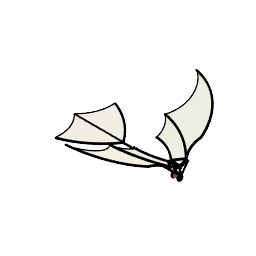
Ornithopter full model (Autodesk Fusion 360 design; units mm, degrees)
Autodesk Fusion 360 part; units mm, degrees
sketch "Sketch1" plane through (0, 0, 0) normal (1, 0, 0) x (0, 1, 0) in component "Component"
  circle A0 centre (0, 0) radius 5
  line L0 (-1, 6.9282) -> (-1, 25)
  arc A1 (1, 25) -> (-1, 25) centre (0, 25) ccw
  line L1 (1, 25) -> (1, 6.9282)
  arc A2 (-1, 6.9282) -> (1, 6.9282) centre (0, 0) ccw
  dimension "d1" = 10
  dimension "d3" = 7
  dimension "d4" = 25
  dimension "d5" = 1
  constraint coincident A0.centre A2.centre
  constraint vertical L0
  constraint tangent L0 A1
  constraint tangent A1 L1
  constraint parallel L0 L1
  constraint concentric A0 A2
  constraint vertical A0.centre A1.centre
  measures "d1" diameter of A0
  measures "d3" radius of A2
  measures "d4" distance of A0.centre A1.centre
  measures "d5" radius of A1
extrude "Extrude1" add sketch "Sketch1" against normal blind 2 makes body 1 in component "Component"
sketch "Sketch2" plane through (0, 0, 0) normal (1, 0, 0) x (0, 1, 0) in component "Component"
  circle A0 centre (0, 0) radius 5
  arc A1 (1, 25) -> (-1, 25) centre (0, 25) ccw
  line L0 (-1, 25) -> (-1, 6.9282)
  arc A2 (-1, 6.9282) -> (1, 6.9282) centre (0, 0) ccw
  line L1 (1, 6.9282) -> (1, 25)
  circle A3 centre (0, 25) radius 1
  dimension "d8" = 2
  constraint concentric A1 A3
  measures "d8" diameter of A3
extrude "Extrude2" add sketch "Sketch2" along normal blind 2 and the other way blind 30 contours A1 A3 bodies 1 in component "Component"
sketch "Sketch3" plane through (-2, 0, 0) normal (-1, 0, 0) x (0, -1, 0) in component "Component"
  arc A0 (-1, 25) -> (1, 25) centre (0, 25) ccw
  line L0 (-1, 25) -> (-1, 6.9282)
  arc A1 (-1, 6.9282) -> (1, 6.9282) centre (0, 0) ccw
  line L1 (1, 6.9282) -> (1, 25)
  circle A2 centre (0, 0) radius 5
  line L2 (1, 7) -> (-1, 7)
  line L3 (-1, 7) -> (-1, 5)
  line L4 (-1, 5) -> (1, 5)
  line L5 (1, 5) -> (1, 7)
  line L6 (1, 7) -> (-1, 5) construction
  line L7 (-1, 7) -> (1, 5) construction
  point P0 (0, 6)
  dimension "d13" = 2
  dimension "d14" = 2
  constraint horizontal L2
  constraint perpendicular L2 L3
  constraint parallel L2 L4
  constraint parallel L3 L5
  constraint coincident L6 P0
  constraint coincident L7 P0
  constraint coincident L1 L2.start
  constraint tangent A2 L4
  measures "d13" distance of L2.start L2.end
  measures "d14" distance of L2.start L4.end
extrude "Extrude4" add sketch "Sketch3" along normal blind 146 contours L0 L1 L2 L3 L4 L5 bodies 1 in component "Component"
ref_plane "WorkPlane1" through (-16, 0, 9) normal (1, 0, 0) x (0, 1, 0) in component "Component"
sketch "Sketch4" plane through (-16, 0, 0) normal (1, 0, 0) x (0, 1, 0) in component "Component"
  circle A0 centre (0, 0) radius 5
  circle A1 centre (0, 0) radius 7
  dimension "d20" = 2
extrude "Extrude5" add sketch "Sketch4" against normal blind 2 bodies 1 in component "Component"
sketch "Sketch5" plane through (-148, 0, 0) normal (-1, 0, 0) x (0, -1, 0) in component "Component"
  line L0 (1, 5) -> (1, 7)
  line L1 (1, 7) -> (-1, 7)
  line L2 (-1, 7) -> (-1, 5)
  line L3 (-1, 5) -> (1, 5)
  line L4 (0.512, 5.5) -> (-0.488, 5.5)
  line L5 (-0.488, 5.5) -> (-0.488, 6.5)
  line L6 (-0.488, 6.5) -> (0.512, 6.5)
  line L7 (0.512, 6.5) -> (0.512, 5.5)
  line L8 (0.512, 5.5) -> (-0.488, 6.5) construction
  line L9 (-0.488, 5.5) -> (0.512, 6.5) construction
  line L10 (1, 7) -> (-1, 7)
  point P0 (0.012, 6)
  dimension "d23" = 1
  dimension "d24" = 1
  dimension "d25" = 0.5
  constraint horizontal L4
  constraint perpendicular L4 L5
  constraint parallel L4 L6
  constraint parallel L5 L7
  constraint coincident L8 P0
  constraint coincident L9 P0
  measures "d23" distance of L4.end L5.end
  measures "d24" distance of L5.end L6.end
  measures "d25" distance of L6 L10
extrude "Extrude6" add sketch "Sketch5" along normal blind 0.7 contours L4 L5 L6 L7 bodies 1 in component "Component"
ref_plane "WorkPlane2" through (-98, 0, -0.0359) normal (-1, 0, 0) x (0, -1, 0) in component "Component"
sketch "Sketch6" plane through (-98, 0, 0) normal (-1, 0, 0) x (0, -1, 0) in component "Component"
  line L0 (-1, 7) -> (1, 7)
  line L1 (1, 7) -> (1, 9)
  line L2 (1, 9) -> (-1, 9)
  line L3 (-1, 9) -> (-1, 7)
  line L4 (-1, 7) -> (1, 9) construction
  line L5 (1, 7) -> (-1, 9) construction
  line L6 (1, 7) -> (-1, 7)
  point P0 (0, 8)
  dimension "d29" = 2
  dimension "d30" = 2
  constraint horizontal L0
  constraint perpendicular L0 L1
  constraint parallel L0 L2
  constraint parallel L1 L3
  constraint coincident L4 P0
  constraint coincident L5 P0
  constraint vertical P0 origin
  constraint collinear L0 L6
  measures "d29" distance of L1.end L2.end
  measures "d30" distance of L0.start L2.end
extrude "Extrude7" add sketch "Sketch6" along normal blind 2 bodies 1 in component "Component"
sketch "Sketch2 (2)" plane through (0, 0, 0) normal (1, 0, 0) x (0, 1, 0) in component "Component'"
  circle A0 centre (0, 0) radius 5
  dimension "d36" = 10
  constraint coincident A0.centre origin
  measures "d36" diameter of A0
extrude "Extrude2'" add sketch "Sketch2 (2)" against normal blind 20 separate body makes body 2 in component "Component'"
sketch "Sketch3 (2)" plane through (0, 0, 0) normal (1, 0, 0) x (0, 1, 0) in component "Component'"
  circle A0 centre (0, 0) radius 5
  circle A1 centre (0, 0) radius 3
  dimension "d39" = 6
  constraint concentric A0 A1
  measures "d39" diameter of A1
extrude "Extrude3" add sketch "Sketch3 (2)" along normal blind 1 contours A1 bodies 2 in component "Component'"
sketch "Sketch4 (2)" plane through (1, 0, 0) normal (1, 0, 0) x (0, 1, 0) in component "Component'"
  circle A0 centre (0, 0) radius 3
  circle A1 centre (0, 0) radius 1
  dimension "d42" = 2
  constraint coincident A0.centre A1.centre
  measures "d42" diameter of A1
extrude "Extrude4'" add sketch "Sketch4 (2)" along normal blind 1 contours A1 bodies 2 in component "Component'"
sketch "Sketch5 (2)" plane through (-20, 0, 0) normal (-1, 0, 0) x (0, -1, 0) in component "Component'"
  circle A0 centre (0, 0) radius 5
  circle A1 centre (-0.6, 4) radius 0.5
  dimension "d45" = 0.6
  dimension "d46" = 4
  dimension "d47" = 1
  measures "d45" horizontal distance of A0.centre A1.centre
  measures "d46" vertical distance of A0.centre A1.centre
  measures "d47" diameter of A1
ref_plane "WorkPlane1" through (0, 0.6, 0) normal (0, 1, 0) x (0, 0, 1) in component "Component'"
sketch "Sketch6 (2)" plane through (0, 0.6, 0) normal (0, 1, 0) x (1, 0, 0) in component "Component'"
  arc A0 (-100, -4) -> (-20, -4) centre (-60, 1795.5555) ccw
  point P0 (-20, -4)
  point P1 (-20, -4)
  point P2 (-20, -4)
  dimension "d49" = 80
  dimension "d50" = 1800
  constraint coincident P2 P0
  constraint horizontal A0.start P1
  measures "d49" distance of A0.start P1
  measures "d50" radius of A0
sweep "Sweep1" add profiles "Sketch5 (2)" path "Sketch6 (2)" along A0 section 1 contours A1 bodies 2 in component "Component'"
mirror "Mirror1" about plane through (0, 0, 0) normal (0, 1, 0) of "Sweep1" in component "Component'"
sketch "Sketch1 (2)" plane through (1, 0, 0) normal (1, 0, 0) x (0, 1, 0) in component "Component''"
  circle A0 centre (0, 0) radius 1
  circle A1 centre (0, 0) radius 3
  circle A2 centre (0, 0) radius 1
  line L0 (0, 0) -> (0, 10.996) construction
  line L1 (0, 0) -> (-5.8821, 10.1881) construction
  circle A3 centre (-2.5, 4.3301) radius 1
  line L2 (-2.5, 2.3301) -> (-1.7321, 1)
  line L3 (-0.7679, 3.3301) -> (0, 2)
  arc A4 (-0.7679, 3.3301) -> (-2.5, 2.3301) centre (-2.5, 4.3301) ccw
  arc A5 (-1.7321, 1) -> (0, 2) centre (0, 0) ccw
  dimension "d59" = 2
  dimension "d60" = 4
  dimension "d61" = 30
  dimension "d62" = 2
  dimension "d63" = 4
  dimension "d64" = 5
  dimension "d65" = 1
  dimension "d66" = 1
  constraint concentric A0 A2
  constraint concentric A2 A5
  constraint coincident A0.centre A1.centre
  constraint vertical L0
  constraint coincident L1 A3.centre
  constraint concentric A3 A4
  constraint parallel L2 L3
  constraint parallel L1 L3
  measures "d59" diameter of A2
  measures "d60" diameter of A5
  measures "d61" angle of L0 L1
  measures "d62" diameter of A3
  measures "d63" diameter of A4
  measures "d64" distance of A0.centre A3.centre
  measures "d65" distance of L1 L2
  measures "d66" distance of L1 L3
extrude "Extrude1'" add sketch "Sketch1 (2)" along normal blind 1 separate body contours A1 L2 L3 A5 | A1 L2 L3 A4 picked at (-1.3017, 1.4521) makes body 3 in component "Component''"
sketch "Sketch1 (3)" plane through (2, 0, 0) normal (1, 0, 0) x (0, 1, 0) in component "Component'''"
  circle A0 centre (-2.5, 4.3301) radius 1
  circle A1 centre (0, 0) radius 1
  arc A2 (-0.7679, 3.3301) -> (-2.5, 2.3301) centre (-2.5, 4.3301) ccw
  line L0 (-2.5, 2.3301) -> (-1.7321, 1)
  arc A3 (-1.7321, 1) -> (0, 2) centre (0, 0) ccw
  line L1 (0, 2) -> (-0.7679, 3.3301)
  circle A4 centre (-2.5, 4.3301) radius 1
  line L2 (-2.5, 4.3301) -> (-2.5, 29.3301) construction
  line L3 (-2.5, 4.3301) -> (21.0114, 36.6908) construction
  circle A5 centre (18.0725, 32.6457) radius 1
  line L4 (16.2454, 31.8322) -> (-2.2909, 6.3192)
  line L5 (-0.6729, 5.1436) -> (17.8634, 30.6567)
  arc A6 (-2.2909, 6.3192) -> (-0.6729, 5.1436) centre (-2.5, 4.3301) ccw
  arc A7 (17.8634, 30.6567) -> (16.2454, 31.8322) centre (18.0725, 32.6457) ccw
  dimension "d70" = 25
  dimension "d71" = 40
  dimension "d72" = 36
  dimension "d73" = 2
  dimension "d75" = 35
  dimension "d76" = 1
  dimension "d77" = 1
  dimension "d78" = 2
  constraint coincident A0.centre A2.centre
  constraint vertical L2
  constraint coincident L3 A5.centre
  constraint coincident A2 L4.end
  constraint coincident A2 L5.start
  constraint parallel L3 L4
  constraint parallel L3 L5
  constraint concentric A4 A6
  constraint concentric A5 A7
  measures "d70" distance of A0.centre L2.end
  measures "d71" distance of A0.centre L3.end
  measures "d72" angle of L2 L3
  measures "d73" diameter of A5
  measures "d75" distance of A0.centre A5.centre
  measures "d76" distance of L3 L4
  measures "d77" distance of L3 L5
  measures "d78" radius of A7
extrude "Extrude1''" add sketch "Sketch1 (3)" along normal blind 1 separate body contours A2 A6 | A2 L4 L5 A7 makes body 4 in component "Component'''"
sketch "Sketch1 (4)" plane through (0, 0, 0) normal (1, 0, 0) x (0, 1, 0) in component "Component''''"
  arc A0 (-1, 25) -> (1, 25) centre (0, 25) ccw
  line L0 (-1, 25) -> (-1, 6.9282)
  arc A1 (-1, 6.9282) -> (1, 6.9282) centre (0, 0) ccw
  line L1 (1, 6.9282) -> (1, 25)
  circle A2 centre (0, 0) radius 5
  arc A3 (-1, 25) -> (1, 25) centre (0, 25) ccw
  circle A4 centre (0, 25) radius 1
  circle A5 centre (18.0725, 32.6457) radius 1 construction
  line L2 (18.0725, 32.6457) -> (0, 25) construction
  line L3 (16.0877, 32.8918) -> (1.2055, 26.5958)
  line L4 (16.8669, 31.0499) -> (1.9848, 24.7539)
  line L5 (1, 24.3373) -> (0.3896, 24.079)
  arc A6 (1.2055, 26.5958) -> (1.9848, 24.7539) centre (0, 25) ccw
  arc A7 (16.8669, 31.0499) -> (16.0877, 32.8918) centre (18.0725, 32.6457) ccw
  dimension "d81" = 4
  dimension "d85" = 2
  constraint coincident A5.centre L2.start
  constraint coincident A0.centre A3.centre
  constraint concentric A5 A7
  constraint coincident L1 L5.start
  constraint collinear L4 L5
  constraint concentric A4 A6
  measures "d81" diameter of A7
  measures "d85" radius of A6
extrude "Extrude1'''" add sketch "Sketch1 (4)" along normal blind 1 separate body contours A0 L0 L1 A3 A4 L5 A6 | L0 L1 A4 L3 L4 A6 A7 makes body 5 in component "Component''''"
sketch "Sketch2 (3)" plane through (1, 0, 0) normal (1, 0, 0) x (0, 1, 0) in component "Component''''"
  arc A0 (1, 25) -> (0.3896, 24.079) centre (0, 25) ccw
  line L0 (1, 25) -> (1, 24.3373)
  line L1 (1, 24.3373) -> (0.3896, 24.079)
  arc A1 (16.8669, 31.0499) -> (16.0877, 32.8918) centre (18.0725, 32.6457) ccw
  line L2 (16.0877, 32.8918) -> (1.2055, 26.5958)
  arc A2 (1.2055, 26.5958) -> (1.9848, 24.7539) centre (0, 25) ccw
  line L3 (1.9848, 24.7539) -> (16.8669, 31.0499)
  circle A3 centre (18.0725, 32.6457) radius 1
extrude "Extrude2''" add sketch "Sketch2 (3)" along normal blind 2 and the other way blind 5 contours A3 bodies 5 in component "Component''''"
mirror "MirrorComponent1" about plane through (0, 0, 0) normal (0, 0, 1) of bodies 5 makes body 6 in component "Component5(Mirror)"
move_face "OffsetFaces1" offset 2 1 faces at (-4, 17.754, -32.744) on bodies 6 in component "Component5(Mirror)"
sketch "Sketch1 (5)" plane through (3, 0, 0) normal (1, 0, 0) x (0, 1, 0) in component "Component'''''"
  circle A0 centre (-2.5, 4.3301) radius 1
  circle A1 centre (18.0725, 32.6457) radius 1
  arc A2 (17.8634, 30.6567) -> (16.2454, 31.8322) centre (18.0725, 32.6457) ccw
  line L0 (16.2454, 31.8322) -> (-2.2909, 6.3192)
  arc A3 (-2.2909, 6.3192) -> (-0.6729, 5.1436) centre (-2.5, 4.3301) ccw
  line L1 (-0.6729, 5.1436) -> (17.8634, 30.6567)
  circle A4 centre (-18.0725, 32.6457) radius 1 construction
  line L2 (-2.5, 4.3301) -> (-18.0725, 32.6457) construction
  line L3 (-2.4584, 6.3297) -> (-16.3616, 31.6099)
  line L4 (-4.2109, 5.3659) -> (-18.1141, 30.6462)
  arc A5 (-4.2109, 5.3659) -> (-2.4584, 6.3297) centre (-2.5, 4.3301) ccw
  arc A6 (-16.3616, 31.6099) -> (-18.1141, 30.6462) centre (-18.0725, 32.6457) ccw
  circle A7 centre (-18.0725, 32.6457) radius 1
  dimension "d93" = 4
  dimension "d94" = 4
  constraint coincident A0.centre A3.centre
  constraint coincident A4.centre L2.end
  measures "d93" diameter of A5
  measures "d94" diameter of A6
extrude "Extrude1''''" add sketch "Sketch1 (5)" along normal blind 1 separate body contours A3 A5 | A3 L3 L4 A6 makes body 7 in component "Component'''''"
sketch "Sketch2 (4)" plane through (3, 0, 0) normal (-1, 0, 0) x (0, -1, 0) in component "Component'''''"
  circle A0 centre (18.0725, 32.6457) radius 1
  circle A1 centre (2.5, 4.3301) radius 1
  arc A2 (2.4584, 6.3297) -> (4.2109, 5.3659) centre (2.5, 4.3301) ccw
  line L0 (4.2109, 5.3659) -> (18.1141, 30.6462)
  arc A3 (18.1141, 30.6462) -> (16.3616, 31.6099) centre (18.0725, 32.6457) ccw
  line L1 (16.3616, 31.6099) -> (2.4584, 6.3297)
  circle A4 centre (2.5, 4.3301) radius 1
  dimension "d99" = 2
  constraint concentric A1 A4
  measures "d99" diameter of A4
extrude "Extrude2'''" add sketch "Sketch2 (4)" along normal blind 2 and the other way blind 1 contours A1 A4 bodies 7 in component "Component'''''"
sketch "Sketch1 (6)" plane through (-100, 0, 0) normal (-1, 0, 0) x (0, -1, 0) in component "Component''''''"
  line L0 (1, 9) -> (-1, 9)
  line L1 (-1, 9) -> (-1, 7)
  line L2 (-1, 7) -> (1, 7)
  line L3 (1, 7) -> (1, 9)
  line L4 (1, 6.9282) -> (1, 25)
  line L5 (-1, 25) -> (-1, 6.9282)
  line L6 (1, 10) -> (-1, 10)
  line L7 (-1, 10) -> (-3.9568, 6.4762)
  line L8 (-3.9568, 6.4762) -> (-3.9568, 1.9762)
  arc A0 (-3.9568, 1.9762) -> (3.9568, 1.9762) centre (0, 1.9762) ccw
  line L9 (3.9568, 1.9762) -> (3.9568, 6.4762)
  line L10 (3.9568, 6.4762) -> (1, 10)
  line L11 (-1, 7) -> (-1, 5)
  line L12 (-1, 5) -> (1, 5)
  line L13 (1, 5) -> (1, 7)
  line L14 (1, 7) -> (-1, 7)
  line L15 (0.512, 6.5) -> (-0.488, 6.5)
  line L16 (0.512, 5.5) -> (0.512, 6.5)
  line L17 (0.512, 6.5) -> (-0.488, 6.5)
  line L18 (-0.488, 6.5) -> (-0.488, 5.5)
  line L19 (-0.488, 5.5) -> (0.512, 5.5)
  line L20 (0.512, 5.5) -> (0.512, 6.5)
  line L21 (-0.488, 6.5) -> (-0.488, 5.5)
  line L22 (-0.488, 5.5) -> (0.512, 5.5)
  dimension "d104" = 130
  dimension "d105" = 130
  dimension "d106" = 4.6
  dimension "d107" = 4.5
  dimension "d108" = 1
  constraint coincident L4 L6.start
  constraint coincident L5 L6.end
  constraint perpendicular L5 L6
  constraint tangent L8 A0
  constraint tangent A0 L9
  constraint vertical origin A0.centre
  constraint vertical L8
  constraint vertical L9
  measures "d104" angle of L6 L7
  measures "d105" angle of L6 L10
  measures "d106" distance of L6.end L7.end
  measures "d107" vertical distance of L7.end L8.end
  measures "d108" distance of L0 L6
extrude "Extrude1'''''" add sketch "Sketch1 (6)" along normal blind 26 separate body contours L0 L1 L2 L3 L4 L5 L14 | L1 L3 L4 L5 L7 L8 A0 L9 L10 L11 L12 L13 | L0 L4 L5 L6 makes body 8 in component "Component''''''"
sketch "Sketch2 (5)" plane through (-100, 0, 0) normal (1, 0, 0) x (0, 1, 0) in component "Component''''''"
  line L0 (-1, 7) -> (1, 7)
  line L1 (1, 7) -> (1, 5)
  line L2 (1, 5) -> (-1, 5)
  line L3 (-1, 5) -> (-1, 7)
  line L4 (-1, 10) -> (-3.9568, 6.4762)
  line L5 (-3.9568, 6.4762) -> (-3.9568, 1.9762)
  arc A0 (-3.9568, 1.9762) -> (3.9568, 1.9762) centre (0, 1.9762) ccw
  line L6 (3.9568, 1.9762) -> (3.9568, 6.4762)
  line L7 (3.9568, 6.4762) -> (1, 10)
  line L8 (1, 10) -> (-1, 10)
  line L9 (1.5, 3.5) -> (-1.5, 3.5)
  line L10 (-1.5, 3.5) -> (-1.5, 5)
  line L11 (-1.5, 5) -> (1.5, 5)
  line L12 (1.5, 5) -> (1.5, 3.5)
  line L13 (1.5, 3.5) -> (-1.5, 5) construction
  line L14 (-1.5, 3.5) -> (1.5, 5) construction
  line L15 (1, 5) -> (-1, 5)
  point P0 (0, 4.25)
  dimension "d111" = 3
  dimension "d112" = 1.5
  constraint horizontal L9
  constraint perpendicular L9 L10
  constraint parallel L9 L11
  constraint parallel L10 L12
  constraint coincident L13 P0
  constraint coincident L14 P0
  constraint vertical P0 origin
  constraint collinear L11 L15
  measures "d111" distance of L10.end L11.end
  measures "d112" distance of L9.start L11.end
extrude "Extrude2''''" add sketch "Sketch2 (5)" along normal blind 5 contours L2 L9 L10 L11 L12 L15 bodies 8 in component "Component''''''"
ref_plane "WorkPlane1" through (-124, 0, 4.0097) normal (-1, 0, 0) x (0, -1, 0) in component "Component''''''"
sketch "Sketch3 (3)" plane through (-124, 0, 0) normal (-1, 0, 0) x (0, -1, 0) in component "Component''''''"
  arc A0 (-3.9568, 1.9762) -> (3.9568, 1.9762) centre (0, 1.9762) ccw
  arc A1 (-2.9568, -0.6532) -> (-2, -0.2599) centre (-2.594, -0.1753) ccw
  line L0 (-3.9568, 6.4762) -> (-3.9568, 1.9762)
  line L1 (0, 0) -> (0, -3.7388) construction
  arc A2 (2, -0.2599) -> (2.9568, -0.6532) centre (2.594, -0.1753) ccw
  arc A3 (2, -0.2599) -> (-2, -0.2599) centre (0, 1.9762) ccw
  dimension "d116" = 6
  dimension "d117" = 2
  dimension "d118" = 0.6
  dimension "d119" = 1
  constraint concentric A0 A3
  constraint coincident A0 A1.start
  constraint coincident L1.start origin
  constraint vertical L1
  constraint symmetric A1.end L1 A2.start
  constraint symmetric A1.start L1 A2.end
  constraint symmetric A1 L1 A2
  measures "d116" diameter of A3
  measures "d117" horizontal distance of L1.start A1.end
  measures "d118" radius of A1
  measures "d119" distance of A1.start L0
extrude "Extrude3'" cut sketch "Sketch3 (3)" against normal blind 20 bodies 8 in component "Component''''''"
sketch "Sketch2 (6)" plane through (-124, 0, 0) normal (1, 0, 0) x (0, 1, 0) in component "Component'''''''"
  arc A0 (-2.9568, -0.6532) -> (2.9568, -0.6532) centre (0, 1.9762) ccw
  arc A1 (2, -0.2599) -> (2.9568, -0.6532) centre (2.594, -0.1753) ccw
  arc A2 (2, -0.2599) -> (-2, -0.2599) centre (0, 1.9762) ccw
  arc A3 (-2.9568, -0.6532) -> (-2, -0.2599) centre (-2.594, -0.1753) ccw
  circle A4 centre (0, 1.9762) radius 3
  dimension "d123" = 6
  constraint concentric A0 A4
  measures "d123" diameter of A4
extrude "Extrude1''''''" add sketch "Sketch2 (6)" along normal blind 20 separate body contours A2 A4 makes body 9 in component "Component'''''''"
fillet "Fillet1" radius 1 1 edges at (-104, -2.797, 0.8913) on bodies 9 in component "Component'''''''"
sketch "Sketch1 (7)" plane through (0, 0, 7) normal (0, 0, 1) x (-1, 0, 0) in component "Component''''''''"
  line L0 (100, 1) -> (100, -1)
  line L1 (100, -1) -> (148, -1)
  line L2 (148, -1) -> (148, 1)
  line L3 (148, 1) -> (100, 1)
  line L4 (148, -1) -> (153, -1)
  arc A0 (153, -1) -> (255.4695, -81) centre (333.5754, 124.6684) ccw
  line L5 (255.4695, -81) -> (256.1796, -79.1303)
  line L6 (148.733, 0.0712) -> (305.2417, 0.0712) construction
  line L7 (155.3919, -0.9288) -> (285.3919, -0.9288)
  arc A1 (154.6416, 0.1424) -> (154.6912, 0.0712) centre (333.5754, 124.6684) ccw
  arc A2 (155.3919, -0.9288) -> (256.1796, -79.1303) centre (333.5754, 124.6684) ccw
  line L8 (285.3919, -0.9288) -> (285.3919, 0.9303)
  line L9 (155.3919, 1.0712) -> (285.3919, 1.0712)
  arc A3 (255.4695, 81.1424) -> (153, 1.1424) centre (333.5754, -124.5259) ccw
  arc A4 (256.1796, 79.2727) -> (155.3919, 1.0712) centre (333.5754, -124.5259) ccw
  line L10 (255.4695, 81.1424) -> (256.1796, 79.2727)
  line L11 (148, 1.1424) -> (153, 1.1424)
  line L12 (285.3919, 1.0712) -> (285.3919, -0.7879)
  line L13 (148, 1.1424) -> (148, -1)
  dimension "d128" = 5
  dimension "d129" = 130
  dimension "d130" = 80
  dimension "d131" = 220
  dimension "d133" = 130
  dimension "d134" = 1
  dimension "d135" = 2
  dimension "d136" = 2
  constraint coincident L1.end L2.start
  constraint perpendicular L2 L4
  constraint horizontal L6
  constraint coincident L7.start A1
  constraint parallel L4 L7
  constraint concentric A0 A1
  constraint coincident L6 A1.end
  constraint concentric A1 A2
  constraint perpendicular L7 L8
  constraint symmetric L1.end L6 L11.start
  constraint symmetric L4.end L6 A3.end
  constraint symmetric A0.end L6 A3.start
  constraint symmetric A0 L6 A3
  constraint symmetric L5.end L6 A4.start
  constraint symmetric L6 L7.start L9.start
  constraint symmetric L6 L7.end L9.end
  constraint symmetric L6 A2 A4
  constraint symmetric L6 L8.end L12.end
  measures "d128" distance of L1.end L4.end
  measures "d129" distance of L4.end A0.end
  measures "d130" vertical distance of L4.end A0.end
  measures "d131" radius of A0
  measures "d133" distance of L7.start L7.end
  measures "d134" distance of L6 L7.end
  measures "d135" distance of A0.end L5.end
  measures "d136" distance of A0 A2
extrude "Extrude1'''''''" add sketch "Sketch1 (7)" against normal blind 2 separate body contours L2 L4 A0 L5 L7 A2 L8 L9 A3 A4 L10 L11 L12 L13 makes body 10 in component "Component''''''''"
sketch "Sketch2 (7)" plane through (0, 0, 7) normal (0, 0, 1) x (-1, 0, 0) in component "Component''''''''"
  arc A0 (255.4695, 81.1424) -> (153, 1.1424) centre (333.5754, -124.5259) ccw
  line L0 (153, 1.1424) -> (148, 1.1424)
  line L1 (148, 1.1424) -> (148, -1)
  line L2 (148, -1) -> (153, -1)
  arc A1 (153, -1) -> (255.4695, -81) centre (333.5754, 124.6684) ccw
  line L3 (255.4695, -81) -> (256.1796, -79.1303)
  arc A2 (155.3919, -0.9288) -> (256.1796, -79.1303) centre (333.5754, 124.6684) ccw
  line L4 (155.3919, -0.9288) -> (285.3919, -0.9288)
  line L5 (285.3919, -0.9288) -> (285.3919, 1.0712)
  line L6 (285.3919, 1.0712) -> (155.3919, 1.0712)
  arc A3 (256.1796, 79.2727) -> (155.3919, 1.0712) centre (333.5754, -124.5259) ccw
  line L7 (256.1796, 79.2727) -> (255.4695, 81.1424)
  arc A4 (255.4695, 81.1424) -> (153, 1.1424) centre (333.5754, -124.5259) ccw
  arc A5 (153, -1) -> (255.4695, -81) centre (333.5754, 124.6684) ccw
  line L8 (153, 1.1424) -> (150.5, 0.0189)
  line L9 (153, -1) -> (150.5, 0.0189)
  arc A6 (285.3919, 0.0712) -> (255.4695, -81) centre (349.8022, -69.7594) ccw
  arc A7 (255.4695, 81.1424) -> (285.3919, 0.0712) centre (349.8022, 69.9018) ccw
  dimension "d139" = 95
  dimension "d140" = 95
  constraint coincident A0.end L0.start
  constraint coincident L2.end A1.start
  constraint midpoint L5 A6.start
  constraint coincident A1.end L3.start
  constraint coincident A0.start L7.end
  measures "d139" radius of A6
  measures "d140" radius of A7
extrude "Extrude2'''''" add sketch "Sketch2 (7)" along normal blind 1 contours A0 A1 A2 L4 L6 A3 A4 A5 L8 L9 A6 A7 | L6 A3 A7 | A2 L4 A6 bodies 10 in component "Component''''''''"
sketch "Sketch3 (4)" plane through (-148, 0, 0) normal (1, 0, 0) x (0, 1, 0) in component "Component''''''''"
  line L0 (1, 7) -> (-1.1424, 7)
  line L1 (-1.1424, 7) -> (-1.1424, 5)
  line L2 (-1.1424, 5) -> (1, 5)
  line L3 (1, 5) -> (1, 7)
  line L4 (1, 5) -> (1, 7)
  line L5 (1, 7) -> (-1, 7)
  line L6 (0.5, 5.5) -> (0.5, 6.5)
  line L7 (0.5, 6.5) -> (-0.6424, 6.5)
  line L8 (-0.6424, 6.5) -> (-0.6424, 5.5)
  line L9 (-0.6424, 5.5) -> (0.5, 5.5)
  dimension "d143" = -0.5
extrude "Extrude3''" cut sketch "Sketch3 (4)" against normal blind 0.7 contours L6 L7 L8 L9 bodies 10 in component "Component''''''''"
sketch "Sketch1 (8)" plane through (-2, 0, 0) normal (-1, 0, 0) x (0, -1, 0) in component "Component'''''''''"
  circle A0 centre (0, 25) radius 1
  circle A1 centre (-18.0725, 32.6457) radius 1
  circle A2 centre (-18.0725, 32.6457) radius 2
  circle A3 centre (0, 25) radius 2
  dimension "d146" = 1
  dimension "d147" = 1
  measures "d146" distance of A1
  measures "d147" distance of A0
extrude "Extrude1''''''''" add sketch "Sketch1 (8)" along normal blind 2 separate body makes body 11 at (-3.3333, -1.9901, 24.8009) makes body 12 at (-3.3333, 16.0824, 32.4466) in component "Component'''''''''"
ref_plane "WorkPlane1" through (-28, 0, 25) normal (-1, 0, 0) x (0, -1, 0) in component "Component'''''''''"
sketch "Sketch2 (8)" plane through (-28, 0, 0) normal (-1, 0, 0) x (0, -1, 0) in component "Component'''''''''"
  circle A0 centre (0, 25) radius 1
  circle A1 centre (0, 25) radius 2
  dimension "d151" = 1
  measures "d151" distance of A0
extrude "Extrude2''''''" add sketch "Sketch2 (8)" against normal blind 2 separate body makes body 13 in component "Component'''''''''"
sketch "Sketch3 (5)" plane through (0, -9.3605, 22.1258) normal (0, -0.389626, 0.920973) x (1, 0, 0) in component "Component'''''''''"
  line L0 (0, 27.6318) -> (0, 11.4727)
  line L1 (0, 11.4727) -> (1, 11.4727)
  line L2 (1, 11.4727) -> (1, 27.6318)
  line L3 (1, 27.6318) -> (0, 27.6318)
  line L4 (-4, 27.5) -> (-2, 27.5)
  line L5 (-4, 31.3639) -> (-4, 27.3639)
  line L6 (-2, 31.3639) -> (-2, 27.3639)
  line L7 (-2, 11.7406) -> (-2, 7.7406)
  line L8 (-4, 11.7406) -> (-4, 7.7406)
  line L9 (-2, 27.5) -> (-2, 11.5)
  line L10 (-2, 11.5) -> (-30, 11.5)
  line L11 (-30, 11.5) -> (-30, 13.5)
  line L12 (-4, 27.5) -> (-4, 13.5)
  line L13 (-4, 13.5) -> (-26, 13.5)
  line L14 (-4, 30.4829) -> (-2, 30.4829)
  arc A0 (-12, 84.4829) -> (-2, 30.4829) centre (47.6585, 67.6048) ccw
  arc A1 (-12, 84.4829) -> (-132, 200.4829) centre (-150.1274, 61.6614) ccw
  arc A2 (-14.0459, 84.5922) -> (-8.7688, 37.406) centre (47.6585, 67.6048) ccw
  arc A3 (-14.0459, 84.5922) -> (-132.259, 198.4997) centre (-150.1274, 61.6614) ccw
  line L15 (-132.259, 198.4997) -> (-132, 200.4829)
  arc A4 (-8.7688, 37.406) -> (-115, 90) centre (-138.9324, -91.9213) ccw
  arc A5 (-5.9062, 31.538) -> (-114.9889, 87.9811) centre (-138.9324, -91.9213) ccw
  arc A6 (-30, 13.5) -> (-92.0271, 38.0002) centre (-93.3007, -55.9912) ccw
  arc A7 (-28.0616, 14.4351) -> (-92, 40) centre (-93.3007, -55.9912) ccw
  line L16 (-92.0271, 38.0002) -> (-92, 40)
  line L17 (-28.0616, 14.4351) -> (-5.9062, 31.538)
  line L18 (-4, 30.4829) -> (-26, 13.5)
  line L19 (-114.9889, 87.9811) -> (-115, 90)
  dimension "d155" = 11.5
  dimension "d156" = 16
  dimension "d157" = 28
  dimension "d158" = 2
  dimension "d160" = 10
  dimension "d161" = 54
  dimension "d162" = 62
  dimension "d163" = 170
  dimension "d164" = 130
  dimension "d165" = 140
  dimension "d167" = 2
  dimension "d168" = 2
  dimension "d170" = 2
  dimension "d171" = 115
  dimension "d172" = 90
  dimension "d173" = 183.4887
  dimension "d174" = 6.9231
  dimension "d175" = -2
  dimension "d176" = 2
  dimension "d177" = 2
  dimension "d178" = 92
  dimension "d179" = 40
  dimension "d180" = 96
  dimension "d181" = 2
  dimension "d182" = 22
  constraint perpendicular L2 L4
  constraint coincident L4.start L5
  constraint coincident L4.end L6
  constraint coincident L7 L9.end
  constraint perpendicular L10 L11
  constraint vertical L11
  constraint coincident L5 L14.start
  constraint coincident L6 L14.end
  constraint perpendicular L6 L14
  constraint tangent A0 A4
  constraint concentric A0 A2
  constraint concentric A1 A3
  constraint parallel L17 L18
  constraint coincident L11.end A6.start
  measures "d155" vertical distance of origin L9.end
  measures "d156" distance of L4.end L9.end
  measures "d157" distance of L9.end L10.end
  measures "d158" distance of L10.end L11.end
  measures "d160" horizontal distance of L14.end A0.start
  measures "d161" vertical distance of L14.end A0.start
  measures "d162" radius of A0
  measures "d163" vertical distance of L14.end A1.end
  measures "d164" horizontal distance of L14.end A1.end
  measures "d165" radius of A1
  measures "d167" distance of A0 A2
  measures "d168" distance of A1 A3
  measures "d170" distance of A1.end A3.end
  measures "d171" horizontal distance of origin A4.end
  measures "d172" vertical distance of origin A4.end
  measures "d173" radius of A4
  measures "d174" distance of L14 A2.end
  measures "d177" distance of L17 L18
  measures "d178" horizontal distance of origin A7.end
  measures "d179" vertical distance of origin A7.end
  measures "d180" radius of A7
  measures "d181" distance of A6.end A7.end
  measures "d182" distance of L12.end L13.end
extrude "Extrude3'''" add sketch "Sketch3 (5)" against normal blind 2 contours L4 L5 L6 L7 L9 L10 L11 L12 L13 L14 A0 A1 A2 A3 L15 A4 A5 A6 A7 L16 L17 L18 L19 bodies 11 12 13 in component "Component'''''''''"
sketch "Sketch4 (3)" plane through (0, -8.5812, 20.2838) normal (0, 0.389626, -0.920973) x (-1, 0, 0) in component "Component'''''''''"
  line L0 (4, 31.0959) -> (4, 30.4829)
  line L1 (4, 30.4829) -> (26, 13.5)
  line L2 (26, 13.5) -> (4, 13.5)
  line L3 (4, 13.5) -> (4, 27.5)
  line L4 (4, 27.5) -> (2, 27.5)
  line L5 (2, 27.5) -> (2, 11.5)
  line L6 (2, 11.5) -> (30, 11.5)
  line L7 (30, 11.5) -> (30, 13.5)
  arc A0 (92.0271, 38.0002) -> (30, 13.5) centre (93.3007, -55.9912) ccw
  line L8 (92.0271, 38.0002) -> (92, 40)
  arc A1 (92, 40) -> (28.0616, 14.4351) centre (93.3007, -55.9912) ccw
  line L9 (28.0616, 14.4351) -> (5.9062, 31.538)
  arc A2 (114.9889, 87.9811) -> (5.9062, 31.538) centre (138.9324, -91.9213) ccw
  line L10 (114.9889, 87.9811) -> (115, 90)
  arc A3 (115, 90) -> (8.7688, 37.406) centre (138.9324, -91.9213) ccw
  arc A4 (8.7688, 37.406) -> (14.0459, 84.5922) centre (-47.6585, 67.6048) ccw
  arc A5 (132.259, 198.4997) -> (14.0459, 84.5922) centre (150.1274, 61.6614) ccw
  line L11 (132.259, 198.4997) -> (132, 200.4829)
  arc A6 (132, 200.4829) -> (12, 84.4829) centre (150.1274, 61.6614) ccw
  arc A7 (2.4524, 31.0959) -> (12, 84.4829) centre (-47.6585, 67.6048) ccw
  line L12 (2.4524, 31.0959) -> (4, 31.0959)
  line L13 (4, 27.5) -> (4, 31.0959)
  line L14 (4, 13.5) -> (4, 27.5)
  line L15 (26, 13.5) -> (4, 13.5)
  arc A8 (2.4524, 31.0959) -> (12, 84.4829) centre (-47.6585, 67.6048) ccw
  arc A9 (92.0271, 38.0002) -> (30, 13.5) centre (93.3007, -55.9912) ccw
  arc A10 (92.0271, 38.0002) -> (30, 13.5) centre (93.3007, -55.9912) ccw
  arc A11 (92.0271, 38.0002) -> (30, 13.5) centre (93.3007, -55.9912) ccw
  arc A12 (132, 200.4829) -> (12, 84.4829) centre (150.1274, 61.6614) ccw
  line L16 (26, 13.5) -> (30, 13.5)
  line L17 (4, 31.0959) -> (2.4524, 31.0959)
  line L18 (4, 31.0959) -> (4, 27.5)
  arc A13 (132, 200.4829) -> (114.9944, 88.9905) centre (172.3795, 137.2809) ccw
  arc A14 (114.9944, 88.9905) -> (92.0271, 38.0002) centre (146.694, 44.0446) ccw
  dimension "d185" = 75
  dimension "d186" = 55
  constraint coincident L1.end L2.start
  constraint coincident L7.end A0.end
  constraint coincident L0.start L12.end
  constraint coincident A7.start L12.start
  constraint coincident L3.end L4.start
  constraint midpoint L10 A13.end
  constraint coincident L11.end A6.start
  constraint coincident A0.start L8.start
  measures "d185" radius of A13
  measures "d186" radius of A14
extrude "Extrude4''" add sketch "Sketch4 (3)" along normal blind 0.2 separate body contours L0 L1 A0 A1 L9 A2 A3 A4 A5 A6 A7 L12 L13 A8 A9 A10 A11 A12 L16 L17 L18 A13 A14 | L1 L2 L3 L13 L14 L15 L18 | A3 A4 A5 A13 | A1 L9 A2 A14 makes body 14 in component "Component'''''''''"
mirror "MirrorComponent2" about plane through (0, 0, 0) normal (0, 0, 1) of bodies 11 14 makes body 15 at (-12.9465, 26.7466, -37.4012) makes body 16 at (-72.6097, 78.2233, -57.0072) in component "Component11(Mirror)"
component "Component" placed x (1, 0, 0) y (0, 1, 0) z (0, 0, 1) at (0, 0, 0)
component "Component'" placed x (1, 0, 0) y (0, 1, 0) z (0, 0, 1) at (0, 0, 0)
component "Component''" placed x (1, 0, 0) y (0, 1, 0) z (0, 0, 1) at (0, 0, 0)
component "Component'''" placed x (1, 0, 0) y (0, 1, 0) z (0, 0, 1) at (0, 0, 0)
component "Component''''" placed x (1, 0, 0) y (0, 1, 0) z (0, 0, 1) at (0, 0, 0)
component "Component5(Mirror)" placed x (1, 0, 0) y (0, -1, 0) z (0, 0, -1) at (1, 0, 0)
component "Component'''''" placed x (1, 0, 0) y (0, 1, 0) z (0, 0, 1) at (0, 0, 0)
component "Component''''''" placed x (1, 0, 0) y (0, 1, 0) z (0, 0, 1) at (0, 0, 0)
component "Component''''''''" placed x (1, 0, 0) y (0, 1, 0) z (0, 0, 1) at (0, 0, 0)
component "Component'''''''''" placed x (1, 0, 0) y (0, 1, 0) z (0, 0, 1) at (0, 0, 0)
component "Component11(Mirror)" placed x (1, 0, 0) y (0, -1, 0) z (0, 0, -1) at (-2, 0, 0)
component "Component'''''''" placed x (1, 0, 0) y (0, 1, 0) z (0, 0, 1) at (0, 0, 0) in component "Component''''''"
